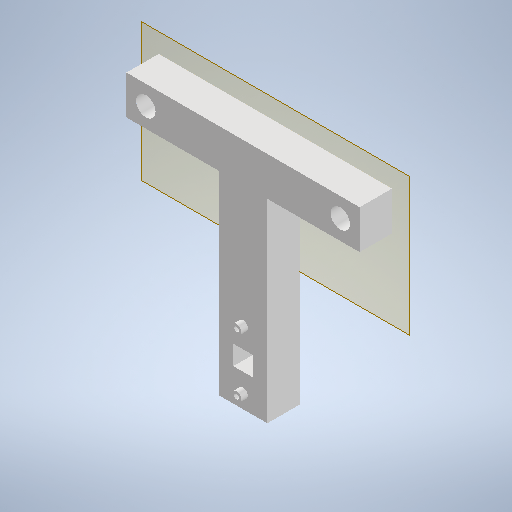
# Autodesk Inventor part: camera_holder
Saved by Autodesk Inventor 2025.1 (Build 291241000, 241)
## iProperties
Created: 2024-11-15
Part Number: camera_holder
Material: Ogólny
Document SubType Name: Modeling
Designer: PC
Density: 1 g/cm^3
Appearance: Domyślna
Author: PC
Autodesk Inventor part; units mm, degrees
ref_plane "YZ Plane" through (0, 0, 0) normal (1, 0, 0) x (0, 1, 0)
ref_plane "XZ Plane" through (0, 0, 0) normal (0, 1, 0) x (-1, 0, 0)
ref_plane "XY Plane" through (0, 0, 0) normal (0, 0, 1) x (1, 0, 0)
ref_plane "Płaszczyzna konstrukcyjna1" through (0, -20, 0) normal (0, 0, 1) x (1, 0, 0)
sketch "Szkic1" plane through (0, -20, 0) normal (0, 0, 1) x (1, 0, 0)
  line L0 (-14.5, -19.3841) -> (-60.5, -19.3841) construction
  line L1 (-14.5, -66.5556) -> (-14.5, -19.3841) projected
  line L2 (-60.5, -66.5556) -> (-14.5, -66.5556) projected
  line L3 (-60.5, -19.3841) -> (-60.5, -66.5556) projected
  line L4 (-62.5, -67.9698) -> (-62.5, -17.9698) projected
  line L5 (-12.5, -67.9698) -> (-62.5, -67.9698) projected
  line L6 (-12.5, -17.9698) -> (-12.5, -67.9698) projected
  line L7 (-62.5, -17.9698) -> (-12.5, -17.9698) construction
  circle A0 centre (-7.5, 10) radius 3 projected
  circle A1 centre (-67.5, 10) radius 3 projected
  line L8 (-75, 0) -> (0, 0) construction
  line L9 (0, 20) -> (0, 0) projected
  line L10 (-75, 20) -> (0, 20) projected
  line L11 (-75, 20) -> (-75, 0) projected
  line L12 (-14.5, -19.3841) -> (-60.5, -66.5556) construction
  line L13 (-60.5, -19.3841) -> (-14.5, -66.5556) construction
  line L14 (-1.5, 16) -> (-73.5, 16)
  line L15 (-73.5, 16) -> (-73.5, 4)
  line L16 (-1.5, 4) -> (-1.5, 16)
  line L17 (-27.5, -27.9698) -> (-47.5, -27.9698) construction
  line L18 (-47.5, -27.9698) -> (-47.5, -57.9698) construction
  line L19 (-47.5, -57.9698) -> (-27.5, -57.9698) construction
  line L20 (-27.5, -57.9698) -> (-27.5, -27.9698) construction
  line L21 (-27.5, -27.9698) -> (-47.5, -57.9698) construction
  line L22 (-47.5, -27.9698) -> (-27.5, -57.9698) construction
  line L23 (-37.5, -27.9698) -> (-37.5, -57.9698) construction
  circle A2 centre (-37.5, -33.6556) radius 0.75
  circle A3 centre (-37.5, -51.6556) radius 0.75
  circle A4 centre (-37.5, -33.6556) radius 1.5
  circle A5 centre (-37.5, -51.6556) radius 1.5
  line L24 (-45, 4) -> (-45, -56)
  line L25 (-45, -56) -> (-30, -56)
  line L26 (-30, -56) -> (-30, 4)
  line L27 (-34.5, -39.9698) -> (-40.5, -39.9698)
  line L28 (-40.5, -39.9698) -> (-40.5, -45.9698)
  line L29 (-40.5, -45.9698) -> (-34.5, -45.9698)
  line L30 (-34.5, -45.9698) -> (-34.5, -39.9698)
  line L31 (-34.5, -39.9698) -> (-40.5, -45.9698) construction
  line L32 (-40.5, -39.9698) -> (-34.5, -45.9698) construction
  line L33 (-73.5, 4) -> (-45, 4)
  line L34 (-30, 4) -> (-1.5, 4)
  line L35 (-37.5, -33.6556) -> (-37.5, -51.6556) construction
  point P0 (-37.5, -42.9698)
  point P1 (-1.5, 10)
  point P2 (-37.5, 4)
  dimension "d0" = 6
  dimension "d1" = 6
  dimension "d2" = 6
  dimension "d3" = 20
  dimension "d4" = 30
  dimension "d5" = 1.5
  dimension "d6" = 18
  dimension "d7" = 3
  dimension "d8" = 3
  dimension "d9" = 6
  dimension "d10" = 6
  dimension "d11" = 15
  dimension "d12" = 60
  dimension "d13" = 4.3444
  constraints: 48 end point, 8 midpoint, 8 parallel, 4 centre point, 4 horizontal, 3 collinear, 3 perpendicular, 2 coincident, 2 point on line, 1 equal radius, 1 horizontal alignment, 1 vertical, 1 vertical alignment
  measures "d0" distance from line of L16 A0.centre
  measures "d1" distance from line of L14 A0.centre
  measures "d2" distance from line of L15 A1.centre
  measures "d3" distance of L19.end L18.end
  measures "d4" distance of L18.end L17.end
  measures "d5" diameter of A2
  measures "d6" distance of A3.centre A2.centre
  measures "d7" diameter of A4
  measures "d8" diameter of A5
  measures "d9" distance of L29.end L27.start
  measures "d10" distance of L28.end L29.end
  measures "d11" distance of L24.end L25.end
  measures "d12" distance of L25.end L26.end
  measures "d13" distance from line of L25 A3.centre
extrude "Wyciągnięcie proste1" add sketch "Szkic1" along normal blind 10 contours L16 L34 L26 L25 L24 L33 L15 L14 | A4 | A5
sketch "Szkic2" plane through (0, -20, 10) normal (0, 0, 1) x (1, 0, 0)
  circle A0 centre (-37.5, -33.6556) radius 1.5 projected
  circle A1 centre (-37.5, -51.6556) radius 1.5 projected
  circle A2 centre (-37.5, -33.6556) radius 0.75 projected
  circle A3 centre (-37.5, -51.6556) radius 0.75 projected
  point P0 (0, 20)
extrude "Wyciągnięcie proste2" add sketch "Szkic2" along normal blind 2
